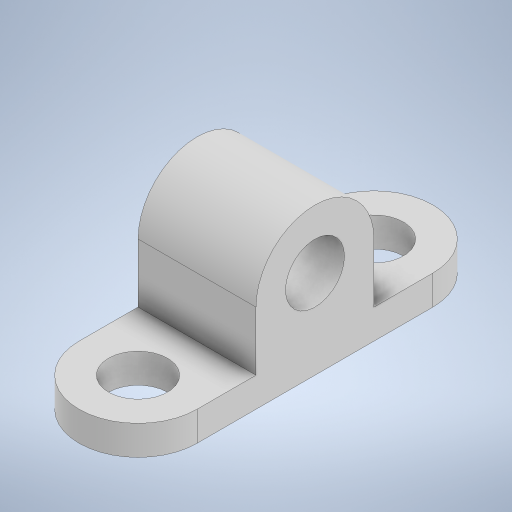
# Autodesk Inventor part: TAREA #1 LAB. DINAMICA CARLOS LUCERO NO.1184321
Saved by Autodesk Inventor 2024 (Build 280153000, 153)
## iProperties
Created: 2024-01-26
Part Number: TAREA #1 LAB. DINAMICA CARLOS LUCERO NO.1184321
Material: Genérico
Document SubType Name: Modeling
Designer: Andres
Density: 1 g/cm^3
Appearance: Valor por defecto
Author: Andres
Autodesk Inventor part; units mm, degrees
ref_plane "YZ Plane" through (0, 0, 0) normal (1, 0, 0) x (0, 1, 0)
ref_plane "XZ Plane" through (0, 0, 0) normal (0, 1, 0) x (-1, 0, 0)
ref_plane "XY Plane" through (0, 0, 0) normal (0, 0, 1) x (1, 0, 0)
sketch "Boceto1" plane through (0, 0, 0) normal (0, 1, 0) x (-1, 0, 0)
  line L0 (-20, 20) -> (-20, -20)
  line L1 (20, -20) -> (20, 20)
  line L2 (-20, 20) -> (20, -20) construction
  line L3 (-20, -20) -> (20, 20) construction
  line L4 (0, 20) -> (0, 40) construction
  line L5 (0, -20) -> (0, -40) construction
  circle A0 centre (0, 40) radius 10
  arc A1 (20, 40) -> (-20, 40) centre (0, 40) ccw
  circle A2 centre (0, -40) radius 10
  arc A3 (-20, -40) -> (20, -40) centre (0, -40) ccw
  line L6 (20, 20) -> (20, 40)
  line L7 (-20, 20) -> (-20, 40)
  line L8 (20, -20) -> (20, -40)
  line L9 (-20, -20) -> (-20, -40)
  point P0 (0, 0)
  dimension "d4" = 20
  dimension "d5" = 40
  dimension "d6" = 20
  dimension "d7" = 40
  constraints: 20 end point, 4 centre point, 4 coincident, 4 point on circle, 3 tangent, 3 vertical, 2 midpoint, 2 point on line, 1 parallel
  measures "d4" diameter of A0
  measures "d5" diameter of A1
  measures "d6" diameter of A2
  measures "d7" diameter of A3
extrude "Extrusión1" add sketch "Boceto1" along normal blind 10
sketch "Boceto2" plane through (20, 0, 40) normal (1, 0, 0) x (0, 0, -1)
  line L0 (80, 10) -> (0, 10) construction
  line L1 (40, 10) -> (40, 30) construction
  arc A0 (60, 30) -> (20, 30) centre (40, 30) ccw
  circle A1 centre (40, 30) radius 10
  line L2 (20, 30) -> (20, 10)
  line L3 (60, 30) -> (60, 10)
  line L4 (20, 10) -> (60, 10)
  point P0 (40, 0)
  dimension "d11" = 40
  dimension "d12" = 20
  constraints: 8 end point, 2 centre point, 2 coincident, 2 midpoint, 2 point on circle, 2 point on line, 2 tangent, 2 vertical, 1 collinear, 1 perpendicular
  measures "d11" diameter of A0
  measures "d12" diameter of A1
extrude "Extrusión2" add sketch "Boceto2" against normal blind 40
